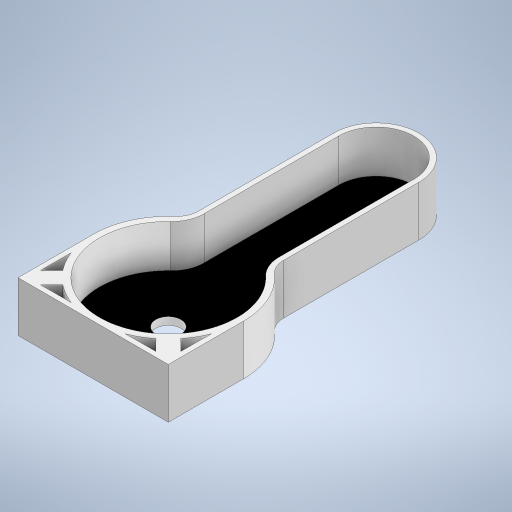
# Autodesk Inventor part: Axel chamber
Saved by Autodesk Inventor 2024 (Build 280153020, 153B)
## iProperties
Created: 2023-09-12
Part Number: Axel chamber
Material: Generic
Document SubType Name: Modeling
Designer: 23also
Density: 1 g/cm^3
Appearance: Default
Author: 23also
Autodesk Inventor part; units mm, degrees
ref_plane "YZ Plane" through (0, 0, 0) normal (1, 0, 0) x (0, 1, 0)
ref_plane "XZ Plane" through (0, 0, 0) normal (0, 1, 0) x (-1, 0, 0)
ref_plane "XY Plane" through (0, 0, 0) normal (0, 0, 1) x (1, 0, 0)
sketch "Sketch2" plane through (0, 0, 0) normal (0, 1, 0) x (-1, 0, 0)
  circle A0 centre (0, 0) radius 30
  dimension "d0" = 60
  constraints: 1 centre point, 1 coincident
  measures "d0" diameter of A0
extrude "Extrusion1" add sketch "Sketch2" along normal blind 20
sketch "Sketch3" plane through (0, 20, 0) normal (0, 1, 0) x (1, 0, 0)
  circle A0 centre (0, 0) radius 27.5
  dimension "d3" = 55
  constraints: 1 centre point, 1 coincident
  measures "d3" diameter of A0
extrude "Extrusion2" cut sketch "Sketch3" against normal blind 17
sketch "Sketch4" plane through (0, 3, 0) normal (0, 1, 0) x (1, 0, 0)
  circle A0 centre (0, 0) radius 5
  dimension "d6" = 10
  constraints: 1 centre point, 1 coincident
  measures "d6" diameter of A0
extrude "Extrusion3" cut sketch "Sketch4" against normal blind 5
sketch "Sketch9" plane through (0, 20, 0) normal (0, 1, 0) x (1, 0, 0)
  line L0 (-15, 35) -> (15, 35)
  line L1 (15, 35) -> (15, 20)
  line L2 (15, 20) -> (-15, 20)
  line L3 (-15, 20) -> (-15, 35)
  circle A0 centre (0, 0) radius 27.5 projected
  line L4 (-15, 35) -> (15, 20) construction
  line L5 (15, 35) -> (-15, 20) construction
  point P0 (0, 27.5)
  constraints: 12 end point, 2 midpoint, 2 parallel, 1 horizontal, 1 perpendicular, 1 vertical alignment, 1 other
extrude "Extrusion6" cut sketch "Sketch9" against normal blind 17 contours L0 L1 A0 L3 | A0 L1 L2 L3 picked at (1.0554, 22.439)
sketch "Sketch10" plane through (0, 20, 0) normal (0, 1, 0) x (1, 0, 0)
  arc A0 (-15, 23.0489) -> (15, 23.0489) centre (0, 0) ccw projected
  line L0 (-15, 23.0489) -> (-17, 23.0489)
  line L1 (-17, 23.0489) -> (-17, 83.0489)
  line L2 (-17, 83.0489) -> (-15, 83.0489)
  line L3 (-15, 83.0489) -> (-15, 23.0489)
  line L4 (15, 25.9808) -> (15, 23.0489) projected
  line L5 (15, 23.0489) -> (17, 23.0489)
  line L6 (17, 23.0489) -> (17, 83.0489)
  line L7 (17, 83.0489) -> (15, 83.0489)
  line L8 (15, 83.0489) -> (15, 23.0489)
  dimension "d17" = 60
  dimension "d18" = 60
  constraints: 16 end point, 4 parallel, 2 horizontal, 2 perpendicular
  measures "d17" distance of L0.end L1.end
  measures "d18" distance of L6.end L5.end
extrude "Extrusion7" add sketch "Sketch10" against normal blind 20
fillet "Fillet1" radius 13 1 edges at (-15, 11.5, -23.0489)
fillet "Fillet2" radius 9 1 edges at (-17, 10, -24.7184)
fillet "Fillet3" radius 13 1 edges at (15, 11.5, -23.0489)
fillet "Fillet4" radius 9 1 edges at (17, 10, -24.7184)
sketch "Sketch12" plane through (0, 0, 0) normal (0, -1, 0) x (1, 0, 0)
  line L0 (-15, -29.2617) -> (-15, -83.0489) projected
  line L1 (15, -25.9808) -> (-15, -25.9808)
  line L2 (-15, -25.9808) -> (-15, -83.0489)
  line L3 (-15, -83.0489) -> (15, -83.0489)
  line L4 (15, -83.0489) -> (15, -25.9808)
  point P0 (0, 0)
  constraints: 8 end point, 2 parallel, 1 horizontal, 1 perpendicular
extrude "Extrusion8" add sketch "Sketch12" against normal blind 3
sketch "Sketch13" plane through (0, 20, 0) normal (0, 1, 0) x (1, 0, 0)
  arc A0 (-20, 22.3607) -> (20, 22.3607) centre (0, 0) ccw projected
  line L0 (30, 0) -> (28, 0)
  line L1 (28, 0) -> (28, -30)
  line L2 (28, -30) -> (30, -30)
  line L3 (30, -30) -> (30, 0)
  line L4 (-30, 0) -> (-28, 0)
  line L5 (-28, 0) -> (-28, -30)
  line L6 (-28, -30) -> (-30, -30)
  line L7 (-30, -30) -> (-30, 0)
  constraints: 16 end point, 4 parallel, 2 horizontal, 2 perpendicular, 2 point on circle
extrude "Extrusion9" add sketch "Sketch13" against normal blind 20
sketch "Sketch14" plane through (0, 20, 0) normal (0, 1, 0) x (1, 0, 0)
  line L0 (-30, -30) -> (-30, 0) projected
  line L1 (30, 0) -> (30, -30) projected
  line L2 (-30, -30) -> (30, -30)
  line L3 (30, -30) -> (30, -28)
  line L4 (30, -28) -> (-30, -28)
  line L5 (-30, -28) -> (-30, -30)
  point P0 (0, 0)
  constraints: 8 end point, 2 parallel, 1 horizontal, 1 perpendicular, 1 point on line
extrude "Extrusion10" add sketch "Sketch14" against normal blind 20
sketch "Sketch17" plane through (28, 0, 10.7703) normal (-1, 0, 0) x (0, 0, 1)
  point P0 (-10.7703, 0)
sketch "Sketch21" plane through (0, 20, 0) normal (0, 1, 0) x (1, 0, 0)
  line L0 (15, 83.0489) -> (-15, 83.0489) projected
  line L1 (-15, 83.0489) -> (-17, 83.0489) projected
  arc A0 (15, 83.0489) -> (-15, 83.0489) centre (0, 82.9999) ccw
  arc A1 (17, 83.0489) -> (-17, 83.0489) centre (0, 82.9999) ccw
  line L2 (-17, 83.0489) -> (-17, 29.0689) projected
  line L3 (-17, 83.0489) -> (-15, 83.0489)
  line L4 (15, 83.0489) -> (17, 83.0489)
  point P0 (0, 0)
  constraints: 4 end point, 4 point on circle, 2 centre point, 1 collinear, 1 concentric, 1 horizontal
extrude "Extrusion15" add sketch "Sketch21" against normal blind 20 contours A0 L1 A1 L4
sketch "Sketch22" plane through (0, 0, 0) normal (0, -1, 0) x (1, 0, 0)
  line L0 (15, -83.0489) -> (15, -25.1247) projected
  arc A0 (-15, -83.0489) -> (15, -83.0489) centre (0, -82.9999) ccw
  line L1 (-15, -83.0489) -> (15, -83.0489) projected
  line L2 (15, -83.0489) -> (-15, -83.0489)
  point P0 (0, 0)
  constraints: 2 end point, 2 point on circle, 1 centre point, 1 horizontal
extrude "Extrusion16" add sketch "Sketch22" against normal blind 3
sketch "Sketch23" plane through (0, 0, 0) normal (0, -1, 0) x (1, 0, 0)
  line L0 (15.995, -25.328) -> (14.0863, -25.328)
  line L1 (14.0863, -25.328) -> (14.0863, -29.7912)
  line L2 (14.0863, -29.7912) -> (15.995, -29.7912)
  line L3 (15.995, -29.7912) -> (15.995, -25.328)
  line L4 (-13.7592, -25.328) -> (-16.454, -25.328)
  line L5 (-16.454, -25.328) -> (-16.454, -29.7912)
  line L6 (-16.454, -29.7912) -> (-13.7592, -29.7912)
  line L7 (-13.7592, -29.7912) -> (-13.7592, -25.328)
  point P0 (0, 0)
  constraints: 16 end point, 4 parallel, 2 horizontal, 2 perpendicular, 2 point on line
extrude "Extrusion17" add sketch "Sketch23" against normal blind 3
sketch "Sketch25" plane through (0, 20, 0) normal (0, 1, 0) x (1, 0, 0)
  line L0 (28, -28) -> (10.7703, -28) projected
  line L1 (28, -28) -> (21.2132, -21.2132)
  arc A0 (10.7703, -28) -> (28, -10.7703) centre (0, 0) ccw projected
  line L2 (28, -28) -> (37.598, -28) construction
  line L3 (28, -28) -> (23, -28)
  line L4 (23, -28) -> (18.5654, -23.5654)
  line L5 (28, -28) -> (28, -23)
  line L6 (28, -23) -> (23.5654, -18.5654)
  line L7 (23.5654, -18.5654) -> (18.5654, -23.5654)
  line L8 (21.2132, -21.2132) -> (21.0654, -21.0654)
  dimension "d53" = 135
  dimension "d54" = 5
  dimension "d55" = 135
  dimension "d56" = 5
  dimension "d57" = 135
  constraints: 16 end point, 4 point on circle, 1 equal length, 1 horizontal, 1 midpoint, 1 perpendicular, 1 point on line, 1 vertical
  measures "d53" angle of L2 L1
  measures "d54" distance of L0.start L3.end
  measures "d55" angle of L3 L4
  measures "d56" distance of L0.start L5.end
  measures "d57" angle of L6 L5
extrude "Extrusion19" add sketch "Sketch25" against normal blind 20 contours L0 L4 A0 L1 | L1 A0 L6 L5
sketch "Sketch27" plane through (0, 20, 0) normal (0, 1, 0) x (1, 0, 0)
  line L0 (-28, -28) -> (-28, -10.7703) projected
  line L1 (-28, -28) -> (-21.2132, -21.2132)
  arc A0 (-28, -10.7703) -> (-10.7703, -28) centre (0, 0) ccw projected
  line L2 (-28, -28) -> (-18.402, -28) construction
  line L3 (-28, -28) -> (-23, -28)
  line L4 (-28, -28) -> (-28, -23)
  line L5 (-28, -23) -> (-23.5654, -18.5654)
  line L6 (-23, -28) -> (-18.5654, -23.5654)
  line L7 (-23, -28) -> (-16.7285, -28) construction
  line L8 (-18.5654, -23.5654) -> (-23.5654, -18.5654)
  dimension "d60" = 45
  dimension "d61" = 5
  dimension "d62" = 5
  dimension "d63" = 135
  dimension "d64" = 45
  constraints: 16 end point, 3 point on circle, 2 equal length, 2 horizontal, 2 point on line
  measures "d60" angle of L2 L1
  measures "d61" distance of L0.start L3.end
  measures "d62" distance of L0.start L4.end
  measures "d63" angle of L4 L5
  measures "d64" angle of L7 L6
extrude "Extrusion20" add sketch "Sketch27" against normal blind 20 contours L0 L5 A0 L1 | L1 A0 L6 L3
body "Solid1"
